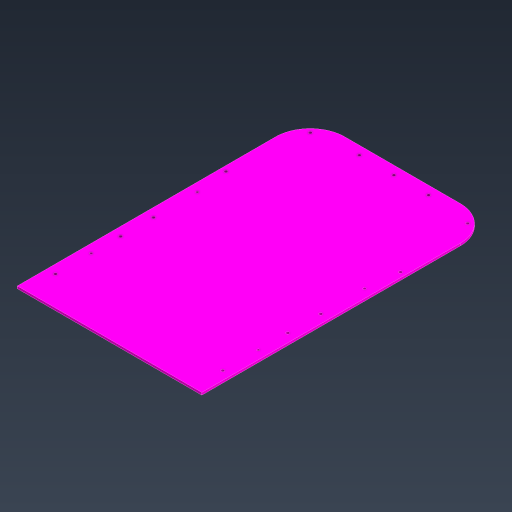
# Autodesk Inventor part: Фанера_крышки
Saved by Autodesk Inventor 2023.2 (Build 272271030, 271C)
## iProperties
Created: 2025-05-05
Part Number: Фанера_крышки
Material: Типовые
Document SubType Name: Modeling
Designer: Олег Коноваленко
Density: 1 g/cm^3
Appearance: Пурпурный
Author: Олег Коноваленко
Autodesk Inventor part; units mm, degrees
ref_plane "YZ Plane" through (0, 0, 0) normal (1, 0, 0) x (0, 1, 0)
ref_plane "XZ Plane" through (0, 0, 0) normal (0, 1, 0) x (-1, 0, 0)
ref_plane "XY Plane" through (0, 0, 0) normal (0, 0, 1) x (1, 0, 0)
sketch "Эскиз1" plane through (0, 0, 0) normal (0, 1, 0) x (-1, 0, 0)
  line L0 (160, -254) -> (-160, -254)
  line L1 (-160, -254) -> (-160, 254)
  line L2 (-160, 254) -> (160, 254)
  line L3 (160, 254) -> (160, -254)
  line L4 (160, -254) -> (-160, 254) construction
  line L5 (-160, -254) -> (160, 254) construction
  arc A0 (-160, -194) -> (-100, -254) centre (-100, -194) ccw
  arc A1 (100, -254) -> (160, -194) centre (100, -194) ccw
  point P0 (0, 0)
  point P1 (0, 0)
  dimension "d0" = 320
  dimension "d1" = 508
  dimension "d8" = 120
  constraints: 12 end point, 4 point on circle, 4 point on line, 4 tangent, 2 centre point, 2 parallel, 1 coincident, 1 equal radius, 1 horizontal, 1 midpoint, 1 perpendicular
  measures "d0" distance between parallel lines of L1 L3
  measures "d1" distance between parallel lines of L2 L0
  measures "d8" diameter of A0
extrude "Выдавливание1" add sketch "Эскиз1" along normal mid plane 4 contours L0 A0 L1 L2 L3 A1
sketch "Эскиз4" plane through (0, -2, 0) normal (0, -1, 0) x (1, 0, 0)
  circle A0 centre (145, 203) radius 2.6 projected
  circle A1 centre (145, 141) radius 2.1 projected
  circle A2 centre (145, 90) radius 2.6 projected
  circle A3 centre (145, 33) radius 2.6 projected
  circle A4 centre (145, -43) radius 2.1 projected
  circle A5 centre (151.2069, -99) radius 2.6 projected
  circle A6 centre (136.3096, -230.3096) radius 2.6 projected
  circle A7 centre (60, -239) radius 2.55 projected
  circle A8 centre (0, -239) radius 2.55 projected
  circle A9 centre (-60, -239) radius 2.55 projected
  circle A10 centre (-136.3096, -230.3096) radius 2.6 projected
  circle A11 centre (-151.2069, -99) radius 2.6 projected
  circle A12 centre (-145, -43) radius 2.1 projected
  circle A13 centre (-145, 33) radius 2.6 projected
  circle A14 centre (-145, 90) radius 2.6 projected
  circle A15 centre (-145, 141) radius 2.1 projected
  circle A16 centre (-145, 203) radius 2.6 projected
  point P0 (0, 0)
extrude "Выдавливание4" cut sketch "Эскиз4" against normal up to next
